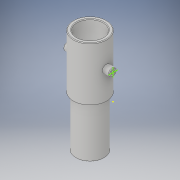
# Autodesk Inventor part: outer_chamber_v6
Saved by Autodesk Inventor 2019 (Build 230136000, 136)
## iProperties
Created: 2021-02-03
Part Number: outer_chamber_v6
Material: Generic
Document SubType Name: Modeling
Designer: wilson
Density: 1 g/cm^3
Appearance: Default
Author: wilson
Autodesk Inventor part; units mm, degrees
ref_plane "YZ Plane" through (0, 0, 0) normal (1, 0, 0) x (0, 1, 0)
ref_plane "XZ Plane" through (0, 0, 0) normal (0, 1, 0) x (-1, 0, 0)
ref_plane "XY Plane" through (0, 0, 0) normal (0, 0, 1) x (1, 0, 0)
sketch "Sketch1" plane through (0, 0, 0) normal (0, 1, 0) x (-1, 0, 0)
  circle A0 centre (0, 0) radius 6.5
  dimension "d0" = 13
  constraints: 1 centre point, 1 coincident
  measures "d0" diameter of A0
extrude "Extrusion1" add sketch "Sketch1" along normal blind 10
sketch "Sketch3" plane through (0, 0, 0) normal (0, -1, 0) x (1, 0, 0)
  circle A0 centre (0, 0) radius 6.5
  dimension "d49" = 13
  constraints: 1 centre point, 1 coincident
  measures "d49" diameter of A0
extrude "Extrusion2" add sketch "Sketch3" along normal blind 1
sketch "Sketch4" plane through (0, -1, 0) normal (0, -1, 0) x (1, 0, 0)
  circle A0 centre (0, 0) radius 5.5
  dimension "d12" = 11
  constraints: 1 centre point, 1 coincident
  measures "d12" diameter of A0
extrude "Extrusion3" add sketch "Sketch4" along normal blind 20
ref_plane "Work Plane2" through (0, 0, 0) normal (0, 1, 0) x (1, 0, 0)
sketch "Sketch5" plane through (0, 0, 0) normal (0, 1, 0) x (1, 0, 0)
  point P0 (0, 0)
  point P1 (0, 0)
  constraints: 1 coincident
hole "Hole2" at (0, 0, 0) direction (0, -1, 0) diameter 9 depth 391.2125 tip angle 118
sketch "Sketch7" plane through (0, 10, 0) normal (0, 1, 0) x (1, 0, 0)
  circle A0 centre (0, 0) radius 6.5
  dimension "d50" = 13
  constraints: 1 centre point, 1 coincident
  measures "d50" diameter of A0
extrude "Extrusion4" add sketch "Sketch7" along normal blind 10
sketch "Sketch9" plane through (0, 0, 0) normal (1, 0, 0) x (0, 1, 0)
  circle A0 centre (10, 0) radius 1.5
  point P0 (0, 0)
  dimension "d32" = 3
  constraints: 1 centre point
  measures "d32" diameter of A0
extrude "Extrusion5" add sketch "Sketch9" along normal mid plane 18
sketch "Sketch10" plane through (0, 0, 0) normal (0, -1, 0) x (1, 0, 0)
  point P0 (0, 0)
  point P1 (0, 0)
  constraints: 1 coincident
hole "Hole4" at (0, 0, 0) direction (0, 1, 0) diameter 10.25 depth 391.2125 tip angle 118
sketch "Sketch11" plane through (9, 10, 0) normal (1, 0, 0) x (0, 0, -1)
  line L0 (-1.6967, 0) -> (1.872, 0)
  line L1 (0, 1.7775) -> (0, -1.6976)
  point P0 (0, -10)
  constraints: 4 end point, 1 horizontal, 1 vertical
sketch "Sketch12" plane through (9, 10, 0) normal (1, 0, 0) x (0, 0, -1)
  point P0 (0, -10)
  point P1 (-0.006, -0.0062)
hole "Hole5" at (9, 9.9938, 0.006) direction (-1, 0, 0) diameter 1 depth 391.2125 tip angle 118
fillet "Fillet1" radius 0.25 3 edges at (0, 20, 5.125) (-6.5, 20, 0) (-5.5, -21, 0)
fillet "Fillet2" radius 0.25 4 edges at (9, 8.5, 0) (-9, 8.5, 0) (9, 9.9938, 0.506) (-9, 9.9938, 0.506)
body "Solid1"
